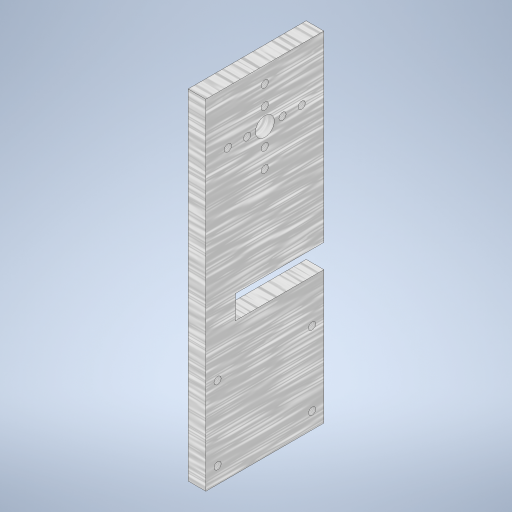
# Autodesk Inventor part: shoulder1_lower_cover
Saved by Autodesk Inventor 2024 (Build 280153000, 153)
## iProperties
Created: 2025-08-06
Part Number: shoulder1_lower_cover
Material: アルミニウム 5052
Document SubType Name: Modeling
Designer: HosodaLab2
Density: 2.68 g/cm^3
Appearance: サテン - ブラシ仕上げ 重厚
個数: 1
Author: HosodaLab2
Autodesk Inventor part; units mm, degrees
ref_plane "YZ Plane" through (0, 0, 0) normal (1, 0, 0) x (0, 1, 0)
ref_plane "XZ Plane" through (0, 0, 0) normal (0, 1, 0) x (-1, 0, 0)
ref_plane "XY Plane" through (0, 0, 0) normal (0, 0, 1) x (1, 0, 0)
sketch "スケッチ1" plane through (0, 0, 0) normal (0, 1, 0) x (-1, 0, 0)
  line L0 (0, 0) -> (-40, 0)
  line L1 (-40, 0) -> (-40, -115)
  line L2 (-40, -115) -> (0, -115)
  line L3 (0, -115) -> (0, 0)
  dimension "d0" = 40
  dimension "d1" = 115
  constraints: 8 end point, 2 parallel, 1 horizontal, 1 perpendicular
  measures "d0" distance of L2.end L1.end
  measures "d1" distance of L1.end L0.end
extrude "押し出し1" add sketch "スケッチ1" along normal blind 6
sketch "スケッチ2" plane through (0, 6, 0) normal (0, 1, 0) x (1, 0, 0)
  line L0 (0, 0) -> (40, 0) construction
  line L1 (20, 0) -> (20, 115) construction
  line L2 (40, 115) -> (0, 115) construction
  point P0 (20, 18)
  dimension "d4" = 18
  constraints: 2 end point, 2 midpoint, 1 point on line
  measures "d4" distance from line of L0 point (20, 18)
hole "穴1" at (20, 6, -18) direction (0, -1, 0) diameter 6.4 end through all
sketch "スケッチ3" plane through (0, 6, 0) normal (0, 1, 0) x (1, 0, 0)
  circle A0 centre (20, 18) radius 3.2 construction
  circle A1 centre (20, 18) radius 12.5 construction
  point P0 (0, 0)
  point P1 (7.5, 18)
  point P2 (20, 5.5)
  point P3 (32.5, 18)
  point P4 (20, 30.5)
  dimension "d12" = 25
  dimension "d15" = 360
  constraints: 1 coincident, 1 horizontal alignment, 7 other
hole "穴2" at (7.5, 6, -18) at (20, 6, -5.5) at (32.5, 6, -18) at (20, 6, -30.5) direction (0, -1, 0) diameter 2.459 end through all thread size "M3x0.5" class "6H" standard "ISO Metric profile"
sketch "スケッチ4" plane through (0, 6, 0) normal (0, 1, 0) x (1, 0, 0)
  line L0 (40, 115) -> (0, 115) construction
  line L1 (0, 115) -> (40, 115) construction
  line L2 (40, 115) -> (40, 110) construction
  line L3 (40, 110) -> (0, 110) construction
  line L4 (0, 110) -> (0, 115) construction
  line L5 (0, 115) -> (0, 0) projected
  line L6 (0, 112.5) -> (40, 112.5) construction
  line L7 (40, 0) -> (40, 115) projected
  line L8 (0, 115) -> (0, 0) construction
  line L9 (40, 85) -> (0, 85) construction
  line L10 (0, 85) -> (0, 90) construction
  line L11 (0, 90) -> (40, 90) construction
  line L12 (40, 90) -> (40, 85) construction
  line L13 (40, 87.5) -> (0, 87.5) construction
  point P0 (4, 112.5)
  point P1 (36, 112.5)
  point P2 (36, 87.5)
  point P3 (4, 87.5)
  dimension "d25" = 5
  dimension "d26" = 4
  dimension "d27" = 4
  dimension "d35" = 5
  dimension "d36" = 25
  constraints: 20 end point, 7 point on line, 4 parallel, 3 midpoint, 2 horizontal, 2 perpendicular
  measures "d25" distance of L1.end L2.end
  measures "d26" distance from line of point (4, 112.5) L5
  measures "d27" distance from line of L7 point (36, 112.5)
  measures "d35" distance of L9.end L10.end
  measures "d36" distance between parallel lines of L0 L11
hole "穴3" [suppressed]
sketch "スケッチ5" plane through (0, 0, 0) normal (0, -1, 0) x (1, 0, 0)
  line L0 (30, -62) -> (0, -62)
  line L1 (0, -62) -> (0, -70)
  line L2 (0, -70) -> (30, -70)
  line L3 (30, -70) -> (30, -62)
  line L4 (0, 0) -> (40, 0) projected
  dimension "d37" = 8
  dimension "d38" = 62
  dimension "d39" = 30
  constraints: 8 end point, 2 parallel, 1 horizontal, 1 perpendicular
  measures "d37" distance between parallel lines of L2 L0
  measures "d38" distance between parallel lines of L4 L0
  measures "d39" distance between parallel lines of L1 L3
extrude "押し出し2" cut sketch "スケッチ5" against normal blind 10
sketch "スケッチ6" plane through (0, 6, 0) normal (0, 1, 0) x (1, 0, 0)
  line L0 (36, 84.5) -> (4, 84.5) construction
  line L1 (4, 84.5) -> (4, 109.5) construction
  line L2 (4, 109.5) -> (36, 109.5) construction
  line L3 (36, 109.5) -> (36, 84.5) construction
  line L4 (40, 0) -> (40, 115) construction
  line L5 (0, 115) -> (0, 70) construction
  line L6 (40, 115) -> (0, 115) construction
  point P0 (0, 0)
  point P1 (20, 109.5)
  dimension "d42" = 4
  dimension "d43" = 4
  dimension "d44" = 5.5
  dimension "d45" = 25
  constraints: 8 end point, 4 coincident, 2 parallel, 1 horizontal, 1 midpoint, 1 perpendicular
  measures "d42" distance between parallel lines of L4 L3
  measures "d43" distance between parallel lines of L5 L1
  measures "d44" distance from line of L6 point (20, 109.5)
  measures "d45" distance between parallel lines of L2 L0
hole "穴4" at (36, 6, -84.5) at (36, 6, -109.5) at (4, 6, -109.5) at (4, 6, -84.5) direction (0, -1, 0) diameter 2.459 end through all thread size "M3x0.5" class "6H" standard "ISO Metric profile"
sketch "スケッチ7" plane through (0, 6, 0) normal (0, 1, 0) x (1, 0, 0)
  circle A0 centre (20, 18) radius 3.2 projected
  circle A1 centre (20, 18) radius 6
  point P0 (0, 0)
  point P1 (20, 12)
  point P2 (14, 18)
  point P3 (20, 24)
  point P4 (26, 18)
  dimension "d53" = 12
  constraints: 4 point on circle, 1 centre point, 1 coincident
  measures "d53" diameter of A1
hole "穴5" at (20, 6, -12) at (14, 6, -18) at (20, 6, -24) at (26, 6, -18) direction (0, -1, 0) diameter 2.459 end through all thread size "M3x0.5" class "6H" standard "ISO Metric profile"
